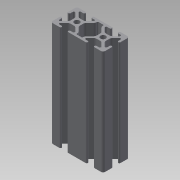
# Autodesk Inventor part: 25-2550
Saved by Autodesk Inventor 2013 (Build 170138000, 138)
## iProperties
Created: 2014-04-23
Part Number: 25-2550
Material: Generic
Document SubType Name: Modeling
Designer: Ross Bowman
Density: 1 g/cm^3
Engineer: Ross Bowman
Catalog Web Link: 8020.net
Vendor: 80/20 Inc.
Company: 80/20 Inc.
Author: Ross Bowman
Keywords: 80/20 , 8020 , T-Slot , Extrusion
Material: 6105-T5 Aluminum
Autodesk Inventor part; units mm, degrees
ref_plane "YZ Plane" through (0, 0, 0) normal (1, 0, 0) x (0, 1, 0)
ref_plane "XZ Plane" through (0, 0, 0) normal (0, 1, 0) x (-1, 0, 0)
ref_plane "XY Plane" through (0, 0, 0) normal (0, 0, 1) x (1, 0, 0)
sketch "Sketch1" plane through (0, 0, 0) normal (0, 0, 1) x (1, 0, 0)
  arc A0 (2.9368, 9.5764) -> (2.1771, 10.36) centre (2.1771, 9.6) ccw
  line L0 (2.9368, 9.5764) -> (2.93, 9.3582)
  arc A1 (2.93, 9.3582) -> (3.8502, 7.1366) centre (6.0718, 9.3582) ccw
  line L1 (7.1715, 3.8153) -> (3.8502, 7.1366)
  arc A2 (8.1, 1.5737) -> (7.1715, 3.8153) centre (4.93, 1.5737) ccw
  line L2 (8.1, -1.5737) -> (8.1, 1.5737)
  arc A3 (7.1715, -3.8153) -> (8.1, -1.5737) centre (4.93, -1.5737) ccw
  line L3 (3.8502, -7.1366) -> (7.1715, -3.8153)
  arc A4 (3.8502, -7.1366) -> (2.93, -9.3582) centre (6.0718, -9.3582) ccw
  line L4 (2.93, -9.3582) -> (2.9368, -9.5764)
  arc A5 (2.1771, -10.36) -> (2.9368, -9.5764) centre (2.1771, -9.6) ccw
  line L5 (2.1771, -10.36) -> (-2.1775, -10.36)
  arc A6 (-2.936, -9.5529) -> (-2.1775, -10.36) centre (-2.1775, -9.6) ccw
  line L6 (-2.93, -9.3582) -> (-2.936, -9.5529)
  arc A7 (-2.93, -9.3582) -> (-3.8502, -7.1366) centre (-6.0718, -9.3582) ccw
  line L7 (-3.8502, -7.1366) -> (-7.1715, -3.8153)
  arc A8 (-8.1, -1.5737) -> (-7.1715, -3.8153) centre (-4.93, -1.5737) ccw
  line L8 (-8.1, -1.5737) -> (-8.1, 1.5737)
  arc A9 (-7.1715, 3.8153) -> (-8.1, 1.5737) centre (-4.93, 1.5737) ccw
  line L9 (-7.1715, 3.8153) -> (-3.8502, 7.1366)
  arc A10 (-3.8502, 7.1366) -> (-2.93, 9.3582) centre (-6.0718, 9.3582) ccw
  line L10 (-2.9368, 9.5764) -> (-2.93, 9.3582)
  arc A11 (-2.1771, 10.36) -> (-2.9368, 9.5764) centre (-2.1771, 9.6) ccw
  line L11 (-2.1771, 10.36) -> (2.1771, 10.36)
  circle A12 centre (-12.5, 0) radius 2.5
  circle A13 centre (12.5, 0) radius 2.5
  line L12 (25, 10.5) -> (25, 4.1733)
  arc A14 (25, 10.5) -> (23, 12.5) centre (23, 10.5) ccw
  line L13 (16.6733, 12.5) -> (23, 12.5)
  arc A15 (16.6733, 12.5) -> (16.6733, 10.36) centre (16.6733, 11.43) ccw
  line L14 (18.9282, 10.36) -> (16.6733, 10.36)
  arc A16 (19.6366, 8.6498) -> (18.9282, 10.36) centre (18.9282, 9.3582) ccw
  line L15 (16.3153, 5.3285) -> (19.6366, 8.6498)
  arc A17 (14.0737, 4.4) -> (16.3153, 5.3285) centre (14.0737, 7.57) ccw
  line L16 (10.9263, 4.4) -> (14.0737, 4.4)
  arc A18 (8.6847, 5.3285) -> (10.9263, 4.4) centre (10.9263, 7.57) ccw
  line L17 (5.3634, 8.6498) -> (8.6847, 5.3285)
  arc A19 (6.0718, 10.36) -> (5.3634, 8.6498) centre (6.0718, 9.3582) ccw
  line L18 (8.3267, 10.36) -> (6.0718, 10.36)
  arc A20 (8.3267, 10.36) -> (8.3267, 12.5) centre (8.3267, 11.43) ccw
  line L19 (8.3267, 12.5) -> (-8.3267, 12.5)
  arc A21 (-8.3267, 12.5) -> (-8.3267, 10.36) centre (-8.3267, 11.43) ccw
  line L20 (-8.3267, 10.36) -> (-6.0718, 10.36)
  arc A22 (-5.3634, 8.6498) -> (-6.0718, 10.36) centre (-6.0718, 9.3582) ccw
  line L21 (-5.3634, 8.6498) -> (-8.6847, 5.3285)
  arc A23 (-10.9263, 4.4) -> (-8.6847, 5.3285) centre (-10.9263, 7.57) ccw
  line L22 (-10.9263, 4.4) -> (-14.0737, 4.4)
  arc A24 (-16.3153, 5.3285) -> (-14.0737, 4.4) centre (-14.0737, 7.57) ccw
  line L23 (-16.3153, 5.3285) -> (-19.6366, 8.6498)
  arc A25 (-18.9282, 10.36) -> (-19.6366, 8.6498) centre (-18.9282, 9.3582) ccw
  line L24 (-18.9282, 10.36) -> (-16.6733, 10.36)
  arc A26 (-16.6733, 10.36) -> (-16.6733, 12.5) centre (-16.6733, 11.43) ccw
  line L25 (-16.6733, 12.5) -> (-23, 12.5)
  arc A27 (-23, 12.5) -> (-25, 10.5) centre (-23, 10.5) ccw
  line L26 (-25, 10.5) -> (-25, 4.1733)
  arc A28 (-25, 4.1733) -> (-22.86, 4.1733) centre (-23.93, 4.1733) ccw
  line L27 (-22.86, 4.1733) -> (-22.86, 6.4282)
  arc A29 (-21.1498, 7.1366) -> (-22.86, 6.4282) centre (-21.8582, 6.4282) ccw
  line L28 (-21.1498, 7.1366) -> (-17.8285, 3.8153)
  arc A30 (-16.9, 1.5737) -> (-17.8285, 3.8153) centre (-20.07, 1.5737) ccw
  line L29 (-16.9, 1.5737) -> (-16.9, -1.5737)
  arc A31 (-17.8285, -3.8153) -> (-16.9, -1.5737) centre (-20.07, -1.5737) ccw
  line L30 (-17.8285, -3.8153) -> (-21.1498, -7.1366)
  arc A32 (-22.86, -6.4282) -> (-21.1498, -7.1366) centre (-21.8582, -6.4282) ccw
  line L31 (-22.86, -6.4282) -> (-22.86, -4.1733)
  arc A33 (-22.86, -4.1733) -> (-25, -4.1733) centre (-23.93, -4.1733) ccw
  line L32 (-25, -4.1733) -> (-25, -10.5)
  arc A34 (-25, -10.5) -> (-23, -12.5) centre (-23, -10.5) ccw
  line L33 (-23, -12.5) -> (-16.6733, -12.5)
  arc A35 (-16.6733, -12.5) -> (-16.6733, -10.36) centre (-16.6733, -11.43) ccw
  line L34 (-16.6733, -10.36) -> (-18.9282, -10.36)
  arc A36 (-19.6366, -8.6498) -> (-18.9282, -10.36) centre (-18.9282, -9.3582) ccw
  line L35 (-19.6366, -8.6498) -> (-16.3153, -5.3285)
  arc A37 (-14.0737, -4.4) -> (-16.3153, -5.3285) centre (-14.0737, -7.57) ccw
  line L36 (-14.0737, -4.4) -> (-10.9263, -4.4)
  arc A38 (-8.6847, -5.3285) -> (-10.9263, -4.4) centre (-10.9263, -7.57) ccw
  line L37 (-8.6847, -5.3285) -> (-5.3634, -8.6498)
  arc A39 (-6.0718, -10.36) -> (-5.3634, -8.6498) centre (-6.0718, -9.3582) ccw
  line L38 (-6.0718, -10.36) -> (-8.3267, -10.36)
  arc A40 (-8.3267, -10.36) -> (-8.3267, -12.5) centre (-8.3267, -11.43) ccw
  line L39 (-8.3267, -12.5) -> (8.3267, -12.5)
  arc A41 (8.3267, -12.5) -> (8.3267, -10.36) centre (8.3267, -11.43) ccw
  line L40 (6.0718, -10.36) -> (8.3267, -10.36)
  arc A42 (5.3634, -8.6498) -> (6.0718, -10.36) centre (6.0718, -9.3582) ccw
  line L41 (8.6847, -5.3285) -> (5.3634, -8.6498)
  arc A43 (10.9263, -4.4) -> (8.6847, -5.3285) centre (10.9263, -7.57) ccw
  line L42 (14.0737, -4.4) -> (10.9263, -4.4)
  arc A44 (16.3153, -5.3285) -> (14.0737, -4.4) centre (14.0737, -7.57) ccw
  line L43 (19.6366, -8.6498) -> (16.3153, -5.3285)
  arc A45 (18.9282, -10.36) -> (19.6366, -8.6498) centre (18.9282, -9.3582) ccw
  line L44 (16.6733, -10.36) -> (18.9282, -10.36)
  arc A46 (16.6733, -10.36) -> (16.6733, -12.5) centre (16.6733, -11.43) ccw
  line L45 (23, -12.5) -> (16.6733, -12.5)
  arc A47 (23, -12.5) -> (25, -10.5) centre (23, -10.5) ccw
  line L46 (25, -4.1733) -> (25, -10.5)
  arc A48 (25, -4.1733) -> (22.86, -4.1733) centre (23.93, -4.1733) ccw
  line L47 (22.86, -6.4282) -> (22.86, -4.1733)
  arc A49 (21.1498, -7.1366) -> (22.86, -6.4282) centre (21.8582, -6.4282) ccw
  line L48 (17.8285, -3.8153) -> (21.1498, -7.1366)
  arc A50 (16.9, -1.5737) -> (17.8285, -3.8153) centre (20.07, -1.5737) ccw
  line L49 (16.9, 1.5737) -> (16.9, -1.5737)
  arc A51 (17.8285, 3.8153) -> (16.9, 1.5737) centre (20.07, 1.5737) ccw
  line L50 (21.1498, 7.1366) -> (17.8285, 3.8153)
  arc A52 (22.86, 6.4282) -> (21.1498, 7.1366) centre (21.8582, 6.4282) ccw
  line L51 (22.86, 4.1733) -> (22.86, 6.4282)
  arc A53 (22.86, 4.1733) -> (25, 4.1733) centre (23.93, 4.1733) ccw
  point P0 (0, 0)
  constraints: 104 end point, 104 point on circle, 54 centre point
extrude "Extrusion1" add sketch "Sketch1" against normal blind 100
body "Solid1"
